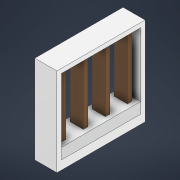
# Autodesk Inventor part: 110033226_ipt_29_城堡四圓塔的窗戶
Saved by Autodesk Inventor 2022 (Build 260153000, 153)
## iProperties
Created: 2022-06-24
Part Number: 110033226_ipt_29_城堡四圓塔的窗戶
Material: 一般
Document SubType Name: Modeling
Designer: User
Density: 1 g/cm^3
Appearance: 預設
Author: User
Autodesk Inventor part; units mm, degrees
ref_plane "YZ Plane" through (0, 0, 0) normal (1, 0, 0) x (0, 1, 0)
ref_plane "XZ Plane" through (0, 0, 0) normal (0, 1, 0) x (-1, 0, 0)
ref_plane "XY Plane" through (0, 0, 0) normal (0, 0, 1) x (1, 0, 0)
sketch "草圖1" plane through (0, 0, 0) normal (0, 1, 0) x (-1, 0, 0)
  line L0 (2.5, 10) -> (-2.5, 10)
  line L1 (-2.5, 10) -> (-2.5, -10)
  line L2 (-2.5, -10) -> (2.5, -10)
  line L3 (2.5, -10) -> (2.5, 10)
  circle A0 centre (0, 7.5) radius 1.7
  circle A1 centre (0, 2.5) radius 1.7
  circle A2 centre (0, -2.5) radius 1.7
  circle A3 centre (0, -7.5) radius 1.7
  point P0 (0, 0)
  point P1 (0, -10)
  point P2 (2.5, 0)
  dimension "d0" = 5
  dimension "d1" = 20
  dimension "d2" = 3.4
  dimension "d3" = 2.5
  dimension "d4" = 2.5
  dimension "d7" = 5
  constraints: 8 end point, 4 centre point, 2 midpoint, 2 parallel, 1 horizontal, 1 horizontal alignment, 1 perpendicular, 1 vertical, 1 vertical alignment, 6 other
  measures "d0" distance of L2.end L1.end
  measures "d1" distance of L1.end L0.end
  measures "d2" diameter of A0
  measures "d3" distance from line of L0 A0.centre
  measures "d4" distance from line of L3 A0.centre
  measures "d7" distance of A0.centre A1.centre
extrude "擠出1" add sketch "草圖1" along normal blind 2 contours L3 L2 L1 L0 | A0 | A1 | A2 | A3
sketch "草圖2" plane through (0, 0, 0) normal (1, 0, 0) x (0, 1, 0)
  line L0 (0, -10) -> (0, 10) projected
  line L1 (0, 10) -> (2, 10) projected
  line L2 (2, -10) -> (2, 10) projected
  line L3 (0, -10) -> (2, -10) projected
  line L4 (0, 10) -> (20, 10)
  line L5 (20, 10) -> (20, -10)
  line L6 (20, -10) -> (0, -10)
  line L7 (0, -10) -> (0, 10)
  line L8 (19, -9) -> (19, 9)
  line L9 (19, 9) -> (1, 9)
  line L10 (1, 9) -> (1, -9)
  line L11 (1, -9) -> (19, -9)
  point P0 (0, 0)
  point P1 (2, 9)
  point P2 (2, -9)
  dimension "d14" = 20
  dimension "d15" = 20
  dimension "d16" = 1
  constraints: 16 end point, 4 parallel, 2 perpendicular, 1 horizontal, 3 other
  measures "d14" distance of L5.end L6.end
  measures "d15" distance of L4.end L5.end
  measures "d16" distance between parallel lines of L5 L8
extrude "擠出2" add sketch "草圖2" along normal mid plane 5 contours L2 L11 L8 L9 L4 L5 L6
sketch "草圖3" plane through (-2.5, 19, -9) normal (0, -1, 0) x (1, 0, 0)
  line L0 (5, 19) -> (0, 19) projected
  line L1 (5, -1) -> (5, 19) projected
  line L2 (0, -1) -> (5, -1) projected
  line L3 (0, 19) -> (0, -1) projected
  line L4 (0, 19) -> (5, 19) projected
  line L5 (5, 19) -> (5, 18) projected
  line L6 (5, 18) -> (0, 18) projected
  line L7 (0, 0) -> (0, 18) projected
  line L8 (0, 0) -> (5, 0) projected
  line L9 (5, 0) -> (5, -1) projected
  line L10 (5, -1) -> (0, -1) projected
  line L11 (0, -1) -> (0, 0) projected
  line L12 (0, 18) -> (0, 19) projected
  line L13 (5, 18) -> (5, 0) projected
  line L14 (1, 17) -> (4, 17)
  line L15 (4, 17) -> (4, 16)
  line L16 (4, 16) -> (1, 16)
  line L17 (1, 16) -> (1, 17)
  line L18 (4, 11) -> (1, 11)
  line L19 (4, 12) -> (4, 11)
  line L20 (1, 12) -> (4, 12)
  line L21 (1, 11) -> (1, 12)
  line L22 (4, 6) -> (1, 6)
  line L23 (4, 7) -> (4, 6)
  line L24 (1, 7) -> (4, 7)
  line L25 (1, 6) -> (1, 7)
  line L26 (4, 1) -> (1, 1)
  line L27 (4, 2) -> (4, 1)
  line L28 (1, 2) -> (4, 2)
  line L29 (1, 1) -> (1, 2)
  point P0 (2.5, 9)
  point P1 (2.5, 17)
  point P2 (2.5, 19)
  point P3 (2.5, 12)
  point P4 (2.5, 7)
  point P5 (2.5, 2)
  dimension "d19" = 3
  dimension "d20" = 1
  dimension "d21" = 1
  dimension "d24" = 5
  constraints: 32 end point, 2 midpoint, 2 parallel, 1 horizontal, 1 perpendicular, 1 vertical, 1 vertical alignment, 27 other
  measures "d19" distance of L15.end L16.end
  measures "d20" distance of L14.end L15.end
  measures "d21" distance between parallel lines of L6 L14
  measures "d24" distance of L15.end L18.start
extrude "擠出3" add sketch "草圖3" along normal up to next separate body contours L14 L15 L16 L17 | L18 L21 L20 L19 | L22 L25 L24 L23 | L26 L29 L28 L27
sketch "草圖4" plane through (0, 2, 0) normal (0, 1, 0) x (1, 0, 0)
  line L0 (2.5, -10) -> (-2.5, -10) projected
  line L1 (-2.5, -10) -> (-2.5, -9) projected
  line L2 (-2.5, -9) -> (2.5, -9) projected
  line L3 (2.5, 9) -> (2.5, -9) projected
  line L4 (2.5, 9) -> (-2.5, 9) projected
  line L5 (-2.5, 9) -> (-2.5, 10) projected
  line L6 (-2.5, 10) -> (2.5, 10) projected
  line L7 (2.5, 10) -> (2.5, 9) projected
  line L8 (2.5, -9) -> (2.5, -10) projected
  line L9 (-2.5, -9) -> (-2.5, 9) projected
  line L10 (1.5, 2) -> (-1.5, 2) projected
  line L11 (-1.5, 2) -> (-1.5, 3) projected
  line L12 (-1.5, 3) -> (1.5, 3) projected
  line L13 (1.5, 3) -> (1.5, 2) projected
  line L14 (1.5, -7) -> (1.5, -8) projected
  line L15 (1.5, -8) -> (-1.5, -8) projected
  line L16 (-1.5, -8) -> (-1.5, -7) projected
  line L17 (-1.5, -7) -> (1.5, -7) projected
  line L18 (1.5, 7) -> (-1.5, 7) projected
  line L19 (-1.5, 7) -> (-1.5, 8) projected
  line L20 (-1.5, 8) -> (1.5, 8) projected
  line L21 (1.5, 8) -> (1.5, 7) projected
  line L22 (-1.5, -3) -> (-1.5, -2) projected
  line L23 (-1.5, -2) -> (1.5, -2) projected
  line L24 (1.5, -2) -> (1.5, -3) projected
  line L25 (1.5, -3) -> (-1.5, -3) projected
  point P0 (0, 0)
extrude "擠出4" add sketch "草圖4" along normal blind 2.5 separate body contours L2 L9 L4 L3
sketch "草圖5" plane through (0, 0, 0) normal (0, -1, 0) x (1, 0, 0)
  line L0 (-2.5, 10) -> (2.5, 10) projected
  line L1 (2.5, 10) -> (2.5, -10) projected
  line L2 (2.5, -10) -> (-2.5, -10) projected
  line L3 (-2.5, -10) -> (-2.5, 10) projected
  circle A0 centre (0, 7.5) radius 1.7
  point P0 (0, 0)
  dimension "d33" = 3.4
  dimension "d34" = 2.5
  dimension "d35" = 2.5
  constraints: 1 centre point
  measures "d33" diameter of A0
  measures "d34" distance from line of L1 A0.centre
  measures "d35" distance from line of L0 A0.centre
extrude "擠出6" cut sketch "草圖5" against normal blind 1.5 contours A0 bodies 1
pattern_linear "矩形陣列2" count 4 spacing 5 along (0, 0, -1) of "擠出6" bodies 1
